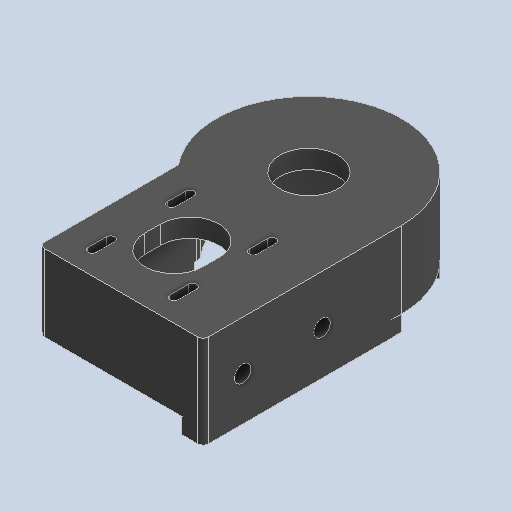
# Autodesk Inventor part: Caja reductora - eje z
Saved by Autodesk Inventor 2026 (Build 300175050, 175E)
## iProperties
Created: 2025-07-23
Part Number: Caja reductora - eje z
Material: Plastico PETG
Document SubType Name: Modeling
Designer: bello
Density: 1.27 g/cm^3
Appearance: Genérico
Author: bello
Autodesk Inventor part; units mm, degrees
ref_plane "YZ Plane" through (0, 0, 0) normal (1, 0, 0) x (0, 1, 0)
ref_plane "XZ Plane" through (0, 0, 0) normal (0, 1, 0) x (-1, 0, 0)
ref_plane "XY Plane" through (0, 0, 0) normal (0, 0, 1) x (1, 0, 0)
sketch "Boceto1" plane through (0, 0, 0) normal (0, 1, 0) x (-1, 0, 0)
  circle A0 centre (0, 0) radius 11
  arc A1 (-35, 0) -> (27, 22.2711) centre (0, 0) ccw
  line L0 (-35, 0) -> (-35, 75)
  line L1 (-35, 75) -> (27, 75)
  line L2 (27, 75) -> (27, 22.2711)
  arc A2 (-11, 45) -> (11, 45) centre (0, 45) ccw
  arc A3 (11, 51) -> (-11, 51) centre (0, 51) ccw
  line L3 (11, 51) -> (11, 45)
  line L4 (-11, 45) -> (-11, 51)
  line L5 (15.5, 66.5) -> (15.5, 59.5) construction
  line L6 (13.95, 66.5) -> (13.95, 59.5)
  line L7 (17.05, 59.5) -> (17.05, 66.5)
  arc A4 (17.05, 66.5) -> (13.95, 66.5) centre (15.5, 66.5) ccw
  arc A5 (13.95, 59.5) -> (17.05, 59.5) centre (15.5, 59.5) ccw
  line L8 (0, 51) -> (0, 45)
  line L9 (0, 48) -> (2.6814, 48)
  line L10 (15.5, 29.5) -> (15.5, 36.5) construction
  line L11 (13.95, 29.5) -> (13.95, 36.5)
  line L12 (17.05, 36.5) -> (17.05, 29.5)
  arc A6 (13.95, 29.5) -> (17.05, 29.5) centre (15.5, 29.5) ccw
  arc A7 (17.05, 36.5) -> (13.95, 36.5) centre (15.5, 36.5) ccw
  line L13 (-15.5, 66.5) -> (-15.5, 59.5) construction
  line L14 (-13.95, 66.5) -> (-13.95, 59.5)
  line L15 (-17.05, 59.5) -> (-17.05, 66.5)
  arc A8 (-13.95, 66.5) -> (-17.05, 66.5) centre (-15.5, 66.5) ccw
  arc A9 (-17.05, 59.5) -> (-13.95, 59.5) centre (-15.5, 59.5) ccw
  line L16 (-13.95, 29.5) -> (-13.95, 36.5)
  line L17 (-15.5, 29.5) -> (-15.5, 36.5) construction
  line L18 (-17.05, 36.5) -> (-17.05, 29.5)
  arc A10 (-17.05, 29.5) -> (-13.95, 29.5) centre (-15.5, 29.5) ccw
  arc A11 (-13.95, 36.5) -> (-17.05, 36.5) centre (-15.5, 36.5) ccw
  point P0 (15.5, 63)
  point P1 (15.5, 33)
  point P2 (-15.5, 63)
  point P3 (-15.5, 33)
  dimension "d0" = 22
  dimension "d1" = 70
  dimension "d2" = 75
  dimension "d3" = 62
  dimension "d4" = 22
  dimension "d5" = 45
  dimension "d6" = 22
  dimension "d7" = 6
  dimension "d8" = 3.1
  dimension "d9" = 7
  dimension "d10" = 15.5
  constraints: 46 end point, 22 point on circle, 21 symmetric about line, 12 centre point, 8 tangent, 3 vertical, 2 coincident, 2 horizontal, 2 midpoint, 1 parallel, 7 other
  measures "d0" diameter of A0
  measures "d1" diameter of A1
  measures "d2" distance of L0.start L0.end
  measures "d3" distance of L0.end L1.end
  measures "d4" diameter of A2
  measures "d5" distance of point (0, 0) L8.end
  measures "d6" diameter of A3
  measures "d7" distance of L8.end L8.start
  measures "d8" diameter of A5
  measures "d9" distance of L7.start L7.end
  measures "d10" horizontal distance of L8.start L5.start
extrude "Extrusión1" add sketch "Boceto1" along normal blind 35
sketch "Boceto3" plane through (0, 0, 0) normal (0, -1, 0) x (1, 0, 0)
  line L0 (-21, 69) -> (21, 69)
  arc A0 (-21, 20) -> (21, 20) centre (0, 0) ccw
  line L1 (-27, 22.2711) -> (-27, 75) projected
  line L2 (-27, 75) -> (35, 75) projected
  line L3 (35, 75) -> (35, 0) projected
  line L4 (-21, 69) -> (-21, 20)
  line L5 (21, 69) -> (21, 20)
  dimension "d15" = 6
  dimension "d17" = 58
  constraints: 6 end point, 2 point on circle, 2 vertical, 1 centre point, 1 coincident, 1 horizontal
  measures "d15" distance between parallel lines of L2 L0
  measures "d17" diameter of A0
extrude "Extrusión2" cut sketch "Boceto3" against normal blind 28
sketch "Boceto4" plane through (0, 0, 0) normal (0, -1, 0) x (1, 0, 0)
  line L0 (-27, 75) -> (35, 75) projected
  line L1 (-27, 22.2711) -> (-27, 75) projected
  line L2 (27, 75) -> (-27, 75)
  line L3 (-27, 75) -> (-27, 69)
  line L4 (-27, 69) -> (27, 69)
  line L5 (27, 69) -> (27, 75)
  line L6 (-21, 69) -> (21, 69) projected
  line L7 (35, 75) -> (35, 0) projected
  line L8 (-20.5061, -20.5061) -> (-24.7487, -24.7487)
  arc A0 (-27, 22.2711) -> (35, 0) centre (0, 0) ccw projected
  line L9 (8.2115, 0) -> (-7.5561, 0)
  line L10 (-27, 22.2711) -> (-21, 22.2711)
  line L11 (-21, 20) -> (-21, 69) projected
  line L12 (-21, 22.2711) -> (-21, 20)
  arc A1 (-27, 22.2711) -> (-24.7487, -24.7487) centre (0, 0) ccw
  line L13 (20.5061, -20.5061) -> (24.7487, -24.7487)
  line L14 (21, 69) -> (21, 20) projected
  line L15 (21, 22.2711) -> (27, 22.2711)
  line L16 (21, 22.2711) -> (21, 20)
  arc A2 (20.5061, -20.5061) -> (21, 20) centre (0, 0) ccw
  arc A3 (24.7487, -24.7487) -> (27, 22.2711) centre (0, 0) ccw
  circle A4 centre (0, 0) radius 11 projected
  line L17 (0, 2.7283) -> (0, -7.844)
  line L18 (7.5058, -28.0118) -> (9.0587, -33.8074)
  line L19 (-7.5058, -28.0118) -> (-9.0587, -33.8074)
  arc A5 (-7.5058, -28.0118) -> (7.5058, -28.0118) centre (0, 0) ccw
  arc A6 (-9.0587, -33.8074) -> (9.0587, -33.8074) centre (0, 0) ccw
  arc A7 (-21, 20) -> (-20.5061, -20.5061) centre (0, 0) ccw
  dimension "d20" = 0
  dimension "d21" = 8
  dimension "d22" = 45
  dimension "d24" = 35
  dimension "d25" = 45
  constraints: 28 end point, 16 point on circle, 6 centre point, 3 horizontal, 3 parallel, 3 point on line, 2 collinear, 2 concentric, 1 perpendicular, 1 vertical
  measures "d20" distance between parallel lines of L6 L4
  measures "d21" distance between parallel lines of L7 L5
  measures "d22" angle of L9 L8
  measures "d24" radius of A1
  measures "d25" angle of L9 L13
extrude "Extrusión3" cut sketch "Boceto4" against normal blind 6 contours L0 L5 L4 L1 | L10 L11 A7 L8 A0 | A0 L13 A2 L14 L15 A3 | L19 A5 L18 A0
sketch "Boceto5" plane through (21, 28, 20) normal (-1, 0, 0) x (0, 0, 1)
  line L0 (49, -22) -> (49, 0) projected
  line L1 (2.2711, -22) -> (49, -22)
  circle A0 centre (10, -11.5) radius 3.1
  circle A1 centre (40, -11.5) radius 3.1
  line L2 (55, -22) -> (55, 7) projected
  line L3 (-20, -22) -> (-20, 7) projected
  point P0 (-20, -28)
  dimension "d30" = 6.2
  dimension "d31" = 30
  dimension "d32" = 15
  dimension "d33" = 10.5
  dimension "d34" = 10.5
  dimension "d50" = 30
  constraints: 2 centre point, 2 end point, 1 equal radius, 1 horizontal
  measures "d30" diameter of A0
  measures "d31" distance of A1.centre A0.centre
  measures "d32" distance from line of L2 A1.centre
  measures "d33" distance from line of L1 A1.centre
  measures "d34" distance from line of L1 A0.centre
  measures "d50" distance from line of L3 A0.centre
extrude "Extrusión4" cut sketch "Boceto5" against normal up to next
sketch "Boceto6" plane through (21, 28, 20) normal (-1, 0, 0) x (0, 0, 1)
  circle A0 centre (40, -11.5) radius 3.1 projected
  line L0 (37.0266, -16.65) -> (34.0533, -11.5)
  line L1 (34.0533, -11.5) -> (37.0266, -6.35)
  line L2 (37.0266, -6.35) -> (42.9734, -6.35)
  line L3 (42.9734, -6.35) -> (45.9467, -11.5)
  line L4 (45.9467, -11.5) -> (42.9734, -16.65)
  line L5 (42.9734, -16.65) -> (37.0266, -16.65)
  circle A1 centre (10, -11.5) radius 3.1 projected
  line L6 (7.0266, -16.65) -> (4.0533, -11.5)
  line L7 (4.0533, -11.5) -> (7.0266, -6.35)
  line L8 (7.0266, -6.35) -> (12.9734, -6.35)
  line L9 (12.9734, -6.35) -> (15.9467, -11.5)
  line L10 (15.9467, -11.5) -> (12.9734, -16.65)
  line L11 (12.9734, -16.65) -> (7.0266, -16.65)
  line L12 (49, -28) -> (2.2711, -28) projected
  point P0 (-20, -28)
  dimension "d37" = 10.3
  constraints: 24 end point, 2 coincident, 2 parallel, 1 collinear, 26 other
  measures "d37" distance between parallel lines of L2 L5
extrude "Extrusión5" cut sketch "Boceto6" against normal blind 4
fillet "Empalme1" radius 2 2 edges at (-27, 20.5, 75) (35, 17.5, 75)
fillet "Empalme2" radius 4 2 edges at (21, 17, 20) (-21, 17, 20)
sketch "Boceto8" plane through (0, 6, 0) normal (0, -1, 0) x (1, 0, 0)
  line L0 (-25, 75) -> (27, 75) projected
  line L1 (27, 75) -> (27, 69) projected
  line L2 (27, 75) -> (27, 69)
  line L3 (27, 69) -> (21, 69)
  line L4 (21, 22.2711) -> (27, 22.2711) projected
  line L5 (21, 69) -> (21, 22.2711)
  line L6 (21, 22.2711) -> (27, 22.2711)
  line L7 (24.7487, -24.7487) -> (20.5061, -20.5061) projected
  line L8 (24.7487, -24.7487) -> (20.5061, -20.5061) projected
  line L9 (20.5061, -20.5061) -> (24.7487, -24.7487)
  line L10 (7.5058, -28.0118) -> (9.0587, -33.8074) projected
  line L11 (7.5058, -28.0118) -> (9.0587, -33.8074)
  line L12 (-9.0587, -33.8074) -> (-7.5058, -28.0118) projected
  line L13 (-7.5058, -28.0118) -> (-9.0587, -33.8074)
  line L14 (-20.5061, -20.5061) -> (-24.7487, -24.7487) projected
  line L15 (-20.5061, -20.5061) -> (-24.7487, -24.7487)
  arc A0 (-27, 22.2711) -> (35, 0) centre (0, 0) ccw projected
  line L16 (-27, 22.2711) -> (-21, 22.2711) projected
  line L17 (-27, 22.2711) -> (-21, 22.2711)
  arc A1 (-27, 22.2711) -> (-24.7487, -24.7487) centre (0, 0) ccw
  arc A2 (-9.0587, -33.8074) -> (9.0587, -33.8074) centre (0, 0) ccw
  arc A3 (24.7487, -24.7487) -> (27, 22.2711) centre (0, 0) ccw
  arc A4 (20.5061, -20.5061) -> (21.9697, 18.9297) centre (0, 0) ccw projected
  arc A5 (7.5058, -28.0118) -> (20.5061, -20.5061) centre (0, 0) ccw
  arc A6 (-20.5061, -20.5061) -> (-7.5058, -28.0118) centre (0, 0) ccw
  circle A7 centre (0, 0) radius 11
  circle A8 centre (0, -32) radius 2 projected
  circle A9 centre (29.8743, 10.8734) radius 2 projected
  circle A10 centre (-29.8743, 10.8734) radius 2 projected
  line L18 (-27, 69) -> (-27, 75)
  line L19 (-27, 69) -> (-27, 73) projected
  line L20 (-27, 75) -> (-25, 75)
  line L21 (-27, 69) -> (-21, 69)
  line L22 (-21, 69) -> (-21, 22.2711)
  line L23 (-21, 21.5407) -> (-21, 69) projected
  line L24 (-27, 22.2711) -> (-21, 22.2711)
  circle A11 centre (0, 72) radius 2 projected
  circle A12 centre (0, 72) radius 2.05
  circle A13 centre (29.8743, 10.8734) radius 2.05
  circle A14 centre (0, -32) radius 2.05
  circle A15 centre (-29.8743, 10.8734) radius 2.05
  dimension "d51" = 6
  dimension "d52" = 46.7289
  dimension "d62" = 4.1
  constraints: 28 end point, 10 centre point, 10 point on circle, 9 collinear, 6 equal radius, 5 coincident, 4 perpendicular, 1 horizontal
  measures "d51" distance of L1.end L3.end
  measures "d52" distance of L3.end L4.start
  measures "d62" diameter of A12
sketch "Boceto10" plane through (0, 6, 0) normal (0, -1, 0) x (1, 0, 0)
  circle A0 centre (0, 72) radius 2.05
  line L0 (6.7845, 0) -> (-6.2714, 0)
  circle A1 centre (0, 0) radius 32
  circle A2 centre (30.0702, 10.9446) radius 2.05
  circle A3 centre (0, -32) radius 2.05
  circle A4 centre (-30.0702, 10.9446) radius 2.05
  circle A5 centre (0, 0) radius 11 projected
  line L1 (0, 0) -> (-30.0702, 10.9446)
  line L2 (0, 0) -> (30.0702, 10.9446)
  line L3 (-25, 75) -> (27, 75) projected
  dimension "d63" = 64
  dimension "d64" = 20
  dimension "d65" = 20
  dimension "d66" = 4.1
  dimension "d69" = 3
  constraints: 6 end point, 5 centre point, 3 equal radius, 3 point on circle, 1 coincident, 1 horizontal
  measures "d63" diameter of A1
  measures "d64" angle of L2 L0
  measures "d65" angle of L0 L1
  measures "d66" diameter of A0
  measures "d69" distance from line of L3 A0.centre
extrude "Extrusión8" cut sketch "Boceto10" against normal blind 5.8 contours A0 | A2 L2 A1 | A1 A2 | A3 A1 | A1 A3 | L2 A2 A1 | A4 A1 | A1 L1 A4 | A4 L1 A1
equation "\"d12\" = Altura"
equation "\"Altura\" = 35"
